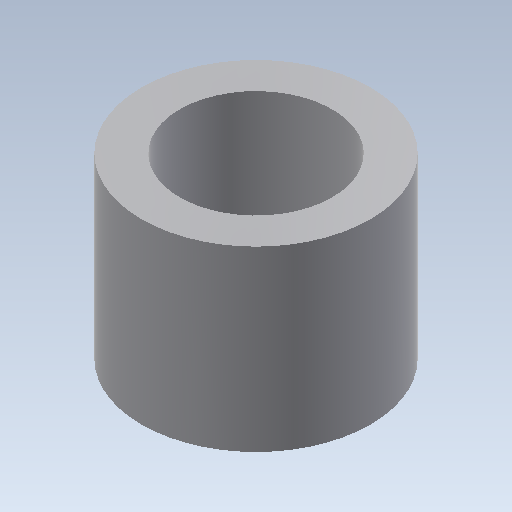
# Autodesk Inventor part: 500-111
Saved by Autodesk Inventor 2020 (Build 240168000, 168)
## iProperties
Created: 2015-04-18
Part Number: 500-111
Material: ABS Plastic
Document SubType Name: Modeling
Designer: Station9
Density: 1.06 g/cm^3
Appearance: Smooth - White
Mass: 0.0327806 g
Surface Area: 1.00138 cm^2
Volume: 0.0309251 cm^3
Author: Station9
Autodesk Inventor part; units mm, degrees
ref_plane "YZ Plane" through (0, 0, 0) normal (1, 0, 0) x (0, 1, 0)
ref_plane "XZ Plane" through (0, 0, 0) normal (0, 1, 0) x (-1, 0, 0)
ref_plane "XY Plane" through (0, 0, 0) normal (0, 0, 1) x (1, 0, 0)
sketch "Sketch1" plane through (0, 0, 0) normal (0, 1, 0) x (-1, 0, 0)
  circle A0 centre (0, 0) radius 2.25
  circle A1 centre (0, 0) radius 1.5
  dimension "d0" = 4.5
  dimension "d1" = 3
  constraints: 2 centre point, 2 coincident
  measures "d0" diameter of A0
  measures "d1" diameter of A1
extrude "Extrusion1" add sketch "Sketch1" along normal blind 3.5
body "Solid1"
